Autodesk Inventor part; units mm, degrees
(part 3 of 10)
  spline S18 degree 5 poles (-4.7205, -4.5819) (-4.7206, -4.5819) (-4.7207, -4.582) (-4.7208, -4.5822) (-4.7211, -4.5824) (-4.7215, -4.5828) (-4.7219, -4.5833) (-4.7224, -4.5838) (-4.723, -4.5844) (-4.7236, -4.585) (-4.7242, -4.5857) (-4.7249, -4.5864) (-4.7257, -4.5872) (-4.7265, -4.5881) (-4.7273, -4.589) (-4.7282, -4.59) (-4.7292, -4.5911) (-4.7302, -4.5922) (-4.7312, -4.5933) (-4.7323, -4.5946) (-4.7335, -4.5958) (-4.7346, -4.5972) (-4.7358, -4.5986) (-4.7371, -4.6) (-4.7384, -4.6015) (-4.7397, -4.6031) (-4.7411, -4.6047) (-4.7425, -4.6064) (-4.744, -4.6081) (-4.7455, -4.6099) (-4.747, -4.6117) (-4.7485, -4.6136) (-4.7501, -4.6156) (-4.7518, -4.6176) (-4.7534, -4.6197) (-4.7555, -4.6222) (-4.7576, -4.6248) (-4.7597, -4.6276) (-4.7626, -4.6313) (-4.7663, -4.6361) (-4.7698, -4.6407) (-4.7734, -4.6455) (-4.777, -4.6504) (-4.7812, -4.6561) (-4.7846, -4.6607) (-4.788, -4.6655) (-4.7915, -4.6705) (-4.796, -4.6769) (-4.7992, -4.6815) (-4.8024, -4.6862) (-4.8057, -4.691) (-4.8104, -4.698) (-4.8142, -4.7038) (-4.8181, -4.7097) (-4.822, -4.7157) (-4.827, -4.7234) (-4.8305, -4.729) (-4.834, -4.7346) (-4.8376, -4.7403) (-4.8422, -4.7478) (-4.8458, -4.7537) (-4.8494, -4.7598) (-4.8531, -4.7659) (-4.8584, -4.7748) (-4.8627, -4.7821) (-4.8669, -4.7895) (-4.8712, -4.7971) (-4.8767, -4.8067) (-4.8805, -4.8135) (-4.8843, -4.8204) (-4.8881, -4.8274) (-4.8931, -4.8366) (-4.897, -4.8438) (-4.9008, -4.8511) (-4.9047, -4.8585) (-4.9097, -4.8682) (-4.9136, -4.8758) (-4.9176, -4.8835) (-4.9221, -4.8924) (-4.9265, -4.9014) (-4.9299, -4.9083) (-4.9333, -4.9152) (-4.9384, -4.9257) (-4.9429, -4.9351) (-4.9474, -4.9447) (-4.9519, -4.9544) (-4.9575, -4.9666) (-4.9615, -4.9753) (-4.9654, -4.9841) (-4.9694, -4.9929) (-4.9745, -5.0044) (-4.9784, -5.0135) (-4.9823, -5.0226) (-4.9862, -5.0318) (-4.9918, -5.0451) (-4.9963, -5.0559) (-5.0008, -5.0668) (-5.0052, -5.0778) (-5.0107, -5.0917) (-5.0146, -5.1015) (-5.0185, -5.1114) (-5.0228, -5.1228) (-5.0272, -5.1344) (-5.0305, -5.1431) (-5.0343, -5.1533) (-5.0381, -5.1636) (-5.0413, -5.1725) (-5.0451, -5.183) (-5.0488, -5.1935) (-5.052, -5.2026) (-5.0557, -5.2133) (-5.0594, -5.2241) (-5.0626, -5.2333) (-5.0662, -5.2442) (-5.0699, -5.2552) (-5.073, -5.2647) (-5.0766, -5.2758) (-5.0801, -5.287) (-5.0832, -5.2967) (-5.0867, -5.308) (-5.0903, -5.3194) (-5.0933, -5.3293) (-5.0967, -5.3408) (-5.1002, -5.3525) (-5.1031, -5.3625) (-5.1066, -5.3742) (-5.1099, -5.3861) (-5.1128, -5.3963) (-5.1162, -5.4082) (-5.1195, -5.4203) (-5.1223, -5.4307) (-5.1256, -5.4428) (-5.1288, -5.4551) (-5.1315, -5.4656) (-5.1347, -5.478) (-5.1379, -5.4904) (-5.1406, -5.5012) (-5.1441, -5.5155) (-5.1476, -5.53) (-5.1506, -5.5427) (-5.154, -5.5574) (-5.1574, -5.5721) (-5.1599, -5.5832) (-5.1632, -5.5981) (-5.1665, -5.613) (-5.1693, -5.6262) (-5.1721, -5.6394) (-5.1757, -5.6565) (-5.1784, -5.6699) (-5.181, -5.6833) (-5.1837, -5.6969) (-5.1863, -5.7104) (-5.1881, -5.7202) (-5.1899, -5.7299) (-5.1917, -5.7397) (-5.1935, -5.7496) (-5.1953, -5.7594) (-5.197, -5.7693) (-5.1987, -5.7793) (-5.2004, -5.7892) (-5.2021, -5.7992) (-5.2038, -5.8092) (-5.2054, -5.8193) (-5.207, -5.8294) (-5.2087, -5.8395) (-5.2102, -5.8496) (-5.2118, -5.8598) (-5.2133, -5.87) (-5.2149, -5.8803) (-5.2164, -5.8905) (-5.2178, -5.9008) (-5.2193, -5.9112) (-5.2207, -5.9215) (-5.2222, -5.9319) (-5.2236, -5.9424) (-5.2249, -5.9528) (-5.2263, -5.9633) (-5.2276, -5.9738) (-5.2289, -5.9844) (-5.231, -6.0013) (-5.2327, -6.0161) (-5.2342, -6.0289) (-5.2354, -6.0396) (-5.2363, -6.0482) knots 0 0 0 0 0 0 0.004167 0.008333 0.0125 0.016667 0.020833 0.025 0.029167 0.033333 0.0375 0.041667 0.045833 0.05 0.054167 0.058333 0.0625 0.066667 0.070833 0.075 0.079167 0.083333 0.0875 0.091667 0.095833 0.1 0.104167 0.108333 0.1125 0.116667 0.120833 0.125 0.129167 0.133333 0.1375 0.141667 0.15 0.154167 0.158333 0.170833 0.183333 0.1875 0.191667 0.195833 0.2125 0.216667 0.220833 0.225 0.2375 0.241667 0.245833 0.25 0.266667 0.270833 0.275 0.279167 0.291667 0.295833 0.3 0.304167 0.316667 0.320833 0.325 0.329167 0.345833 0.35 0.354167 0.358333 0.370833 0.375 0.379167 0.383333 0.395833 0.4 0.404167 0.408333 0.420833 0.425 0.429167 0.4375 0.441667 0.445833 0.45 0.466667 0.470833 0.475 0.479167 0.491667 0.495833 0.5 0.504167 0.516667 0.520833 0.525 0.529167 0.545833 0.55 0.554167 0.558333 0.570833 0.575 0.579167 0.5875 0.591667 0.595833 0.604167 0.608333 0.6125 0.620833 0.625 0.629167 0.6375 0.641667 0.645833 0.654167 0.658333 0.6625 0.670833 0.675 0.679167 0.6875 0.691667 0.695833 0.704167 0.708333 0.7125 0.720833 0.725 0.729167 0.7375 0.741667 0.745833 0.754167 0.758333 0.7625 0.770833 0.775 0.779167 0.791667 0.795833 0.8 0.808333 0.8125 0.816667 0.829167 0.833333 0.8375 0.841667 0.854167 0.858333 0.8625 0.866667 0.870833 0.875 0.879167 0.883333 0.8875 0.891667 0.895833 0.9 0.904167 0.908333 0.9125 0.916667 0.920833 0.925 0.929167 0.933333 0.9375 0.941667 0.945833 0.95 0.954167 0.958333 0.9625 0.966667 0.970833 0.975 0.979167 0.983333 1 1 1 1 1 1
  arc A19 (-5.2363, -6.0482) -> (-4.7314, -6.4509) centre (0, 0) ccw
  spline S19 degree 5 poles (-4.7314, -6.4509) (-4.7253, -6.4488) (-4.7171, -6.4459) (-4.707, -6.4424) (-4.6949, -6.4381) (-4.6808, -6.4331) (-4.6708, -6.4295) (-4.6608, -6.4258) (-4.6508, -6.4222) (-4.6409, -6.4186) (-4.631, -6.4149) (-4.6212, -6.4112) (-4.6114, -6.4075) (-4.6016, -6.4038) (-4.5918, -6.4001) (-4.5821, -6.3963) (-4.5724, -6.3926) (-4.5628, -6.3888) (-4.5532, -6.3851) (-4.5436, -6.3813) (-4.534, -6.3775) (-4.5245, -6.3737) (-4.5151, -6.3698) (-4.5056, -6.366) (-4.4962, -6.3621) (-4.4869, -6.3583) (-4.4775, -6.3544) (-4.4682, -6.3505) (-4.459, -6.3466) (-4.4498, -6.3427) (-4.4406, -6.3388) (-4.4277, -6.3333) (-4.415, -6.3277) (-4.4023, -6.3222) (-4.3898, -6.3166) (-4.3737, -6.3094) (-4.3559, -6.3014) (-4.3383, -6.2933) (-4.3209, -6.2852) (-4.3036, -6.277) (-4.2865, -6.2688) (-4.2745, -6.2631) (-4.2627, -6.2573) (-4.2509, -6.2516) (-4.2359, -6.2441) (-4.2243, -6.2383) (-4.2128, -6.2325) (-4.1997, -6.2258) (-4.1867, -6.2191) (-4.177, -6.2141) (-4.1658, -6.2082) (-4.1547, -6.2023) (-4.1452, -6.1972) (-4.1342, -6.1913) (-4.1233, -6.1854) (-4.114, -6.1803) (-4.1032, -6.1744) (-4.0925, -6.1685) (-4.0834, -6.1634) (-4.0728, -6.1574) (-4.0623, -6.1514) (-4.0534, -6.1463) (-4.043, -6.1404) (-4.0328, -6.1344) (-4.024, -6.1292) (-4.0139, -6.1233) (-4.0039, -6.1173) (-3.9953, -6.1121) (-3.9854, -6.1061) (-3.9756, -6.1002) (-3.9673, -6.095) (-3.9576, -6.089) (-3.948, -6.083) (-3.9398, -6.0779) (-3.9317, -6.0727) (-3.9197, -6.065) (-3.9091, -6.0582) (-3.8986, -6.0514) (-3.8882, -6.0445) (-3.8754, -6.036) (-3.8665, -6.03) (-3.8577, -6.0241) (-3.849, -6.0181) (-3.838, -6.0105) (-3.8294, -6.0045) (-3.821, -5.9986) (-3.8126, -5.9927) (-3.8008, -5.9843) (-3.7915, -5.9776) (-3.7823, -5.9708) (-3.7732, -5.9642) (-3.762, -5.9558) (-3.7542, -5.95) (-3.7465, -5.9442) (-3.7389, -5.9384) (-3.7293, -5.931) (-3.7219, -5.9253) (-3.7146, -5.9196) (-3.7074, -5.9139) (-3.6982, -5.9066) (-3.6912, -5.9009) (-3.6842, -5.8953) (-3.6764, -5.8889) (-3.6687, -5.8825) (-3.663, -5.8778) (-3.6564, -5.8723) (-3.6499, -5.8668) (-3.6444, -5.8621) (-3.638, -5.8567) (-3.6318, -5.8513) (-3.6265, -5.8466) (-3.6204, -5.8413) (-3.6144, -5.836) (-3.6093, -5.8315) (-3.6035, -5.8262) (-3.5977, -5.821) (-3.5929, -5.8166) (-3.5873, -5.8114) (-3.5818, -5.8063) (-3.5771, -5.802) (-3.5718, -5.7969) (-3.5665, -5.792) (-3.5621, -5.7877) (-3.557, -5.7828) (-3.552, -5.778) (-3.5478, -5.7738) (-3.5429, -5.7691) (-3.5382, -5.7643) (-3.5342, -5.7603) (-3.5296, -5.7557) (-3.5251, -5.7511) (-3.5214, -5.7472) (-3.517, -5.7427) (-3.5128, -5.7383) (-3.5092, -5.7346) (-3.5052, -5.7302) (-3.5012, -5.726) (-3.4979, -5.7224) (-3.494, -5.7182) (-3.4903, -5.7141) (-3.4872, -5.7107) (-3.4837, -5.7067) (-3.4802, -5.7028) (-3.4773, -5.6995) (-3.474, -5.6958) (-3.4708, -5.6921) (-3.4681, -5.689) (-3.4655, -5.6859) (-3.4622, -5.6819) (-3.4593, -5.6785) (-3.4565, -5.6752) (-3.4539, -5.6719) (-3.4513, -5.6687) (-3.4495, -5.6665) (-3.4478, -5.6644) (-3.4461, -5.6622) (-3.4445, -5.6602) (-3.4429, -5.6581) (-3.4413, -5.6561) (-3.4398, -5.6542) (-3.4383, -5.6523) (-3.4369, -5.6504) (-3.4356, -5.6486) (-3.4342, -5.6469) (-3.433, -5.6452) (-3.4317, -5.6435) (-3.4306, -5.6419) (-3.4294, -5.6404) (-3.4283, -5.6389) (-3.4273, -5.6374) (-3.4263, -5.6361) (-3.4254, -5.6347) (-3.4245, -5.6335) (-3.4236, -5.6322) (-3.4228, -5.6311) (-3.4221, -5.63) (-3.4213, -5.6289) (-3.4207, -5.628) (-3.4201, -5.627) (-3.4195, -5.6262) (-3.419, -5.6254) (-3.4185, -5.6247) (-3.418, -5.624) (-3.4176, -5.6234) (-3.4172, -5.6228) (-3.417, -5.6223) (-3.4168, -5.622) (-3.4166, -5.6218) (-3.4166, -5.6217) knots -1 -1 -1 -1 -1 -1 -0.9875 -0.983333 -0.979167 -0.975 -0.970833 -0.966667 -0.9625 -0.958333 -0.954167 -0.95 -0.945833 -0.941667 -0.9375 -0.933333 -0.929167 -0.925 -0.920833 -0.916667 -0.9125 -0.908333 -0.904167 -0.9 -0.895833 -0.891667 -0.8875 -0.883333 -0.879167 -0.875 -0.870833 -0.866667 -0.854167 -0.85 -0.845833 -0.841667 -0.829167 -0.8125 -0.808333 -0.804167 -0.8 -0.7875 -0.783333 -0.779167 -0.775 -0.7625 -0.758333 -0.754167 -0.745833 -0.741667 -0.7375 -0.729167 -0.725 -0.720833 -0.7125 -0.708333 -0.704167 -0.695833 -0.691667 -0.6875 -0.679167 -0.675 -0.670833 -0.6625 -0.658333 -0.654167 -0.645833 -0.641667 -0.6375 -0.629167 -0.625 -0.620833 -0.6125 -0.608333 -0.604167 -0.6 -0.583333 -0.579167 -0.575 -0.570833 -0.558333 -0.554167 -0.55 -0.545833 -0.533333 -0.529167 -0.525 -0.520833 -0.504167 -0.5 -0.495833 -0.491667 -0.479167 -0.475 -0.470833 -0.466667 -0.454167 -0.45 -0.445833 -0.441667 -0.429167 -0.425 -0.420833 -0.4125 -0.408333 -0.404167 -0.395833 -0.391667 -0.3875 -0.379167 -0.375 -0.370833 -0.3625 -0.358333 -0.354167 -0.345833 -0.341667 -0.3375 -0.329167 -0.325 -0.320833 -0.3125 -0.308333 -0.304167 -0.295833 -0.291667 -0.2875 -0.279167 -0.275 -0.270833 -0.2625 -0.258333 -0.254167 -0.245833 -0.241667 -0.2375 -0.229167 -0.225 -0.220833 -0.2125 -0.208333 -0.204167 -0.195833 -0.191667 -0.1875 -0.179167 -0.175 -0.170833 -0.166667 -0.154167 -0.15 -0.145833 -0.141667 -0.1375 -0.133333 -0.129167 -0.125 -0.120833 -0.116667 -0.1125 -0.108333 -0.104167 -0.1 -0.095833 -0.091667 -0.0875 -0.083333 -0.079167 -0.075 -0.070833 -0.066667 -0.0625 -0.058333 -0.054167 -0.05 -0.045833 -0.041667 -0.0375 -0.033333 -0.029167 -0.025 -0.020833 -0.016667 -0.0125 -0.008333 0 0 0 0 0 0
  line L37 (-3.4166, -5.6217) -> (-3.4162, -5.6212)
  line L38 (-0.6391, -6.5474) -> (-0.639, -6.5467)
  line L39 (-0.639, -6.5467) -> (-0.5586, -5.7228)
  arc A20 (-0.5586, -5.7228) -> (0.5586, -5.7228) centre (0, 0) ccw
  line L40 (0.5586, -5.7228) -> (0.639, -6.5467)
  line L41 (0.639, -6.5467) -> (0.6391, -6.5474)
  spline S20 degree 5 poles (0.6391, -6.5474) (0.6391, -6.5475) (0.6391, -6.5476) (0.6391, -6.5478) (0.6391, -6.5482) (0.6392, -6.5488) (0.6393, -6.5494) (0.6394, -6.5501) (0.6395, -6.5509) (0.6396, -6.5517) (0.6397, -6.5527) (0.6399, -6.5537) (0.64, -6.5548) (0.6402, -6.556) (0.6404, -6.5572) (0.6406, -6.5585) (0.6408, -6.5599) (0.6411, -6.5614) (0.6413, -6.5629) (0.6416, -6.5645) (0.6419, -6.5662) (0.6422, -6.568) (0.6425, -6.5698) (0.6429, -6.5717) (0.6433, -6.5736) (0.6437, -6.5756) (0.6441, -6.5777) (0.6445, -6.5799) (0.6449, -6.5821) (0.6454, -6.5844) (0.6459, -6.5867) (0.6464, -6.5891) (0.6469, -6.5916) (0.6475, -6.5941) (0.6481, -6.5967) (0.6488, -6.5999) (0.6496, -6.6032) (0.6504, -6.6065) (0.6515, -6.6111) (0.6529, -6.6171) (0.6543, -6.6226) (0.6558, -6.6284) (0.6574, -6.6343) (0.6592, -6.6411) (0.6608, -6.6466) (0.6624, -6.6523) (0.6641, -6.6582) (0.6663, -6.6657) (0.6679, -6.671) (0.6696, -6.6765) (0.6713, -6.682) (0.6738, -6.6901) (0.676, -6.6966) (0.6781, -6.7034) (0.6804, -6.7102) (0.6834, -6.7189) (0.6855, -6.7251) (0.6877, -6.7313) (0.69, -6.7377) (0.6929, -6.746) (0.6953, -6.7525) (0.6978, -6.7591) (0.7003, -6.7658) (0.704, -6.7755) (0.707, -6.7834) (0.7101, -6.7913) (0.7133, -6.7994) (0.7175, -6.8096) (0.7204, -6.8169) (0.7234, -6.8242) (0.7265, -6.8315) (0.7306, -6.8411) (0.7338, -6.8486) (0.7371, -6.8562) (0.7405, -6.8639) (0.7454, -6.8749) (0.7494, -6.8839) (0.7535, -6.8929) (0.7578, -6.902) (0.7631, -6.9135) (0.767, -6.9216) (0.7709, -6.9297) (0.7749, -6.938) (0.7801, -6.9486) (0.7842, -6.957) (0.7884, -6.9654) (0.7927, -6.9738) (0.7983, -6.9848) (0.8027, -6.9933) (0.8072, -7.002) (0.8124, -7.0119) (0.8177, -7.0219) (0.8218, -7.0294) (0.8266, -7.0382) (0.8314, -7.0471) (0.8356, -7.0548) (0.8406, -7.0637) (0.8456, -7.0727) (0.85, -7.0805) (0.8552, -7.0896) (0.8605, -7.0987) (0.865, -7.1066) (0.8704, -7.1158) (0.8758, -7.125) (0.8806, -7.133) (0.8862, -7.1423) (0.8918, -7.1517) (0.8967, -7.1597) (0.9025, -7.1692) (0.9084, -7.1786) (0.9134, -7.1868) (0.9194, -7.1963) (0.9255, -7.2059) (0.9307, -7.2141) (0.9369, -7.2238) (0.9432, -7.2334) (0.9486, -7.2417) (0.955, -7.2515) (0.9615, -7.2612) (0.9671, -7.2696) (0.9737, -7.2794) (0.9804, -7.2893) (0.9861, -7.2978) (0.993, -7.3077) (0.9998, -7.3176) (1.0058, -7.3261) (1.0128, -7.3361) (1.0199, -7.3461) (1.026, -7.3547) (1.0333, -7.3648) (1.0406, -7.3748) (1.0469, -7.3835) (1.0543, -7.3936) (1.0618, -7.4038) (1.0683, -7.4125) (1.0759, -7.4227) (1.0836, -7.4329) (1.0903, -7.4417) (1.0981, -7.4519) (1.1061, -7.4622) (1.1129, -7.471) (1.121, -7.4813) (1.1291, -7.4916) (1.1361, -7.5005) (1.1432, -7.5093) (1.1527, -7.5212) (1.1611, -7.5316) (1.1696, -7.542) (1.1794, -7.5539) (1.1893, -7.5658) (1.1967, -7.5748) (1.2043, -7.5837) (1.2131, -7.5942) (1.2207, -7.6032) (1.2297, -7.6137) (1.2388, -7.6242) (1.2479, -7.6347) (1.2558, -7.6437) (1.2637, -7.6528) (1.2704, -7.6603) (1.2771, -7.6678) (1.2838, -7.6754) (1.2905, -7.6829) (1.2973, -7.6905) (1.3042, -7.698) (1.311, -7.7056) (1.318, -7.7132) (1.3249, -7.7207) (1.3319, -7.7283) (1.3389, -7.7359) (1.346, -7.7434) (1.3531, -7.751) (1.3602, -7.7586) (1.3674, -7.7662) (1.3746, -7.7738) (1.3818, -7.7813) (1.3891, -7.7889) (1.3964, -7.7965) (1.4038, -7.8041) (1.4111, -7.8117) (1.4186, -7.8193) (1.4305, -7.8315) (1.4411, -7.8421) (1.4502, -7.8512) (1.4578, -7.8588) (1.4639, -7.8649) knots 0 0 0 0 0 0 0.004167 0.008333 0.0125 0.016667 0.020833 0.025 0.029167 0.033333 0.0375 0.041667 0.045833 0.05 0.054167 0.058333 0.0625 0.066667 0.070833 0.075 0.079167 0.083333 0.0875 0.091667 0.095833 0.1 0.104167 0.108333 0.1125 0.116667 0.120833 0.125 0.129167 0.133333 0.1375 0.141667 0.15 0.154167 0.158333 0.170833 0.183333 0.1875 0.191667 0.195833 0.2125 0.216667 0.220833 0.225 0.2375 0.241667 0.245833 0.25 0.266667 0.270833 0.275 0.279167 0.291667 0.295833 0.3 0.304167 0.316667 0.320833 0.325 0.329167 0.345833 0.35 0.354167 0.358333 0.370833 0.375 0.379167 0.383333 0.395833 0.4 0.404167 0.408333 0.425 0.429167 0.433333 0.4375 0.45 0.454167 0.458333 0.4625 0.475 0.479167 0.483333 0.4875 0.5 0.504167 0.508333 0.516667 0.520833 0.525 0.533333 0.5375 0.541667 0.55 0.554167 0.558333 0.566667 0.570833 0.575 0.583333 0.5875 0.591667 0.6 0.604167 0.608333 0.616667 0.620833 0.625 0.633333 0.6375 0.641667 0.65 0.654167 0.658333 0.666667 0.670833 0.675 0.683333 0.6875 0.691667 0.7 0.704167 0.708333 0.716667 0.720833 0.725 0.733333 0.7375 0.741667 0.75 0.754167 0.758333 0.766667 0.770833 0.775 0.783333 0.7875 0.791667 0.8 0.804167 0.808333 0.8125 0.825 0.829167 0.833333 0.841667 0.845833 0.85 0.854167 0.8625 0.866667 0.875 0.879167 0.883333 0.8875 0.891667 0.895833 0.9 0.904167 0.908333 0.9125 0.916667 0.920833 0.925 0.929167 0.933333 0.9375 0.941667 0.945833 0.95 0.954167 0.958333 0.9625 0.966667 0.970833 0.975 0.979167 0.983333 1 1 1 1 1 1
  arc A21 (1.4639, -7.8649) -> (2.0935, -7.7212) centre (0, 0) ccw
  spline S21 degree 5 poles (2.0935, -7.7212) (2.0957, -7.7151) (2.0986, -7.707) (2.1021, -7.6968) (2.1063, -7.6847) (2.1112, -7.6705) (2.1146, -7.6605) (2.118, -7.6504) (2.1213, -7.6403) (2.1247, -7.6303) (2.128, -7.6203) (2.1312, -7.6103) (2.1345, -7.6003) (2.1377, -7.5904) (2.1408, -7.5804) (2.144, -7.5705) (2.1471, -7.5606) (2.1501, -7.5507) (2.1532, -7.5408) (2.1562, -7.531) (2.1592, -7.5211) (2.1621, -7.5113) (2.165, -7.5015) (2.1679, -7.4918) (2.1708, -7.482) (2.1736, -7.4723) (2.1764, -7.4626) (2.1791, -7.4529) (2.1818, -7.4432) (2.1845, -7.4336) (2.1877, -7.422) (2.1909, -7.4105) (2.194, -7.399) (2.197, -7.3875) (2.2011, -7.3723) (2.2045, -7.359) (2.2079, -7.3458) (2.2112, -7.3326) (2.2154, -7.3157) (2.2186, -7.3026) (2.2217, -7.2895) (2.2248, -7.2765) (2.2291, -7.258) (2.2324, -7.2433) (2.2357, -7.2286) (2.2388, -7.214) (2.2427, -7.1958) (2.2454, -7.1832) (2.248, -7.1706) (2.2505, -7.158) (2.2537, -7.1419) (2.2561, -7.1295) (2.2584, -7.1171) (2.2607, -7.1048) (2.2639, -7.0872) (2.2664, -7.0733) (2.2688, -7.0594) (2.2711, -7.0456) (2.2739, -7.0284) (2.2758, -7.0165) (2.2776, -7.0046) (2.2794, -6.9928) (2.2817, -6.9777) (2.2833, -6.966) (2.285, -6.9543) (2.2868, -6.9411) (2.2885, -6.928) (2.2897, -6.9182) (2.2911, -6.9068) (2.2925, -6.8954) (2.2936, -6.8858) (2.2949, -6.8746) (2.2961, -6.8634) (2.2971, -6.8539) (2.2983, -6.8429) (2.2993, -6.8319) (2.3002, -6.8226) (2.3012, -6.8117) (2.3022, -6.801) (2.303, -6.7918) (2.3038, -6.7811) (2.3046, -6.7706) (2.3053, -6.7615) (2.3061, -6.7511) (2.3067, -6.7407) (2.3073, -6.7318) (2.3079, -6.7216) (2.3085, -6.7114) (2.3089, -6.7027) (2.3094, -6.6927) (2.3099, -6.6827) (2.3102, -6.6742) (2.3106, -6.6644) (2.3109, -6.6546) (2.3112, -6.6463) (2.3114, -6.6367) (2.3116, -6.6271) (2.3118, -6.619) (2.3119, -6.6096) (2.312, -6.6003) (2.3121, -6.5923) (2.3121, -6.5832) (2.3121, -6.5741) (2.3121, -6.5663) (2.3121, -6.5574) (2.312, -6.5485) (2.3118, -6.541) (2.3117, -6.5323) (2.3115, -6.5237) (2.3113, -6.5163) (2.3111, -6.5078) (2.3108, -6.4995) (2.3105, -6.4924) (2.3102, -6.4841) (2.3098, -6.476) (2.3095, -6.4691) (2.309, -6.4611) (2.3086, -6.4532) (2.3082, -6.4466) (2.3077, -6.4388) (2.3072, -6.4312) (2.3067, -6.4248) (2.3061, -6.4173) (2.3055, -6.41) (2.305, -6.4038) (2.3044, -6.3966) (2.3037, -6.3895) (2.3031, -6.3835) (2.3025, -6.3766) (2.3017, -6.3698) (2.3011, -6.3641) (2.3004, -6.3575) (2.2996, -6.3509) (2.299, -6.3454) (2.2982, -6.3391) (2.2974, -6.3329) (2.2967, -6.3277) (2.2958, -6.3216) (2.295, -6.3157) (2.2943, -6.3107) (2.2934, -6.305) (2.2926, -6.2994) (2.2918, -6.2947) (2.2909, -6.2893) (2.2901, -6.284) (2.2893, -6.2795) (2.2884, -6.2744) (2.2875, -6.2695) (2.2867, -6.2653) (2.286, -6.2612) (2.2852, -6.2572) (2.2843, -6.2526) (2.2834, -6.2482) (2.2825, -6.2439) (2.2816, -6.2397) (2.2808, -6.2356) (2.2801, -6.2328) (2.2795, -6.23) (2.2789, -6.2273) (2.2783, -6.2246) (2.2777, -6.222) (2.2771, -6.2195) (2.2765, -6.2171) (2.2759, -6.2147) (2.2754, -6.2123) (2.2748, -6.2101) (2.2742, -6.2079) (2.2737, -6.2058) (2.2732, -6.2037) (2.2726, -6.2017) (2.2721, -6.1998) (2.2716, -6.198) (2.2711, -6.1962) (2.2706, -6.1945) (2.2702, -6.1928) (2.2697, -6.1913) (2.2693, -6.1898) (2.2689, -6.1883) (2.2685, -6.187) (2.2681, -6.1857) (2.2677, -6.1845) (2.2674, -6.1834) (2.267, -6.1823) (2.2667, -6.1813) (2.2664, -6.1804) (2.2662, -6.1796) (2.2659, -6.1788) (2.2657, -6.1782) (2.2654, -6.1774) (2.2653, -6.1769) (2.2652, -6.1766) (2.2651, -6.1764) (2.265, -6.1763) knots -1 -1 -1 -1 -1 -1 -0.9875 -0.983333 -0.979167 -0.975 -0.970833 -0.966667 -0.9625 -0.958333 -0.954167 -0.95 -0.945833 -0.941667 -0.9375 -0.933333 -0.929167 -0.925 -0.920833 -0.916667 -0.9125 -0.908333 -0.904167 -0.9 -0.895833 -0.891667 -0.8875 -0.883333 -0.879167 -0.875 -0.870833 -0.8625 -0.858333 -0.854167 -0.85 -0.8375 -0.833333 -0.829167 -0.825 -0.8125 -0.808333 -0.804167 -0.8 -0.783333 -0.779167 -0.775 -0.770833 -0.758333 -0.754167 -0.75 -0.745833 -0.733333 -0.729167 -0.725 -0.720833 -0.704167 -0.7 -0.695833 -0.691667 -0.679167 -0.675 -0.670833 -0.666667 -0.654167 -0.65 -0.645833 -0.6375 -0.633333 -0.629167 -0.620833 -0.616667 -0.6125 -0.604167 -0.6 -0.595833 -0.5875 -0.583333 -0.579167 -0.570833 -0.566667 -0.5625 -0.554167 -0.55 -0.545833 -0.5375 -0.533333 -0.529167 -0.520833 -0.516667 -0.5125 -0.504167 -0.5 -0.495833 -0.4875 -0.483333 -0.479167 -0.470833 -0.466667 -0.4625 -0.454167 -0.45 -0.445833 -0.4375 -0.433333 -0.429167 -0.420833 -0.416667 -0.4125 -0.404167 -0.4 -0.395833 -0.3875 -0.383333 -0.379167 -0.370833 -0.366667 -0.3625 -0.354167 -0.35 -0.345833 -0.3375 -0.333333 -0.329167 -0.320833 -0.316667 -0.3125 -0.304167 -0.3 -0.295833 -0.2875 -0.283333 -0.279167 -0.270833 -0.266667 -0.2625 -0.254167 -0.25 -0.245833 -0.2375 -0.233333 -0.229167 -0.220833 -0.216667 -0.2125 -0.204167 -0.2 -0.195833 -0.1875 -0.183333 -0.179167 -0.175 -0.170833 -0.158333 -0.154167 -0.15 -0.145833 -0.141667 -0.1375 -0.133333 -0.129167 -0.125 -0.120833 -0.116667 -0.1125 -0.108333 -0.104167 -0.1 -0.095833 -0.091667 -0.0875 -0.083333 -0.079167 -0.075 -0.070833 -0.066667 -0.0625 -0.058333 -0.054167 -0.05 -0.045833 -0.041667 -0.0375 -0.033333 -0.029167 -0.025 -0.020833 -0.016667 -0.0125 -0.008333 0 0 0 0 0 0
  line L42 (2.265, -6.1763) -> (2.2648, -6.1757)
  line L43 (2.2648, -6.1757) -> (1.9798, -5.3984)
  arc A22 (1.9798, -5.3984) -> (2.9863, -4.9137) centre (0, 0) ccw
  line L44 (4.7205, -4.5819) -> (4.72, -4.5814)
  line L45 (4.72, -4.5814) -> (4.126, -4.0048)
  spline S22 degree 5 poles (5.2363, -6.0482) (5.2356, -6.0418) (5.2347, -6.0332) (5.2335, -6.0225) (5.232, -6.0098) (5.2302, -5.9949) (5.2289, -5.9844) (5.2276, -5.9738) (5.2263, -5.9633) (5.2249, -5.9528) (5.2236, -5.9424) (5.2222, -5.9319) (5.2207, -5.9215) (5.2193, -5.9112) (5.2178, -5.9008) (5.2164, -5.8905) (5.2149, -5.8803) (5.2133, -5.87) (5.2118, -5.8598) (5.2102, -5.8496) (5.2087, -5.8395) (5.207, -5.8294) (5.2054, -5.8193) (5.2038, -5.8092) (5.2021, -5.7992) (5.2004, -5.7892) (5.1987, -5.7793) (5.197, -5.7693) (5.1953, -5.7594) (5.1935, -5.7496) (5.1917, -5.7397) (5.1892, -5.726) (5.1866, -5.7124) (5.1841, -5.6988) (5.1814, -5.6853) (5.178, -5.668) (5.1741, -5.6489) (5.1702, -5.6299) (5.1661, -5.6111) (5.162, -5.5925) (5.1578, -5.5739) (5.1549, -5.561) (5.1519, -5.5482) (5.1489, -5.5355) (5.145, -5.5191) (5.1419, -5.5065) (5.1388, -5.494) (5.1352, -5.4798) (5.1315, -5.4656) (5.1288, -5.4551) (5.1256, -5.4428) (5.1223, -5.4307) (5.1195, -5.4203) (5.1162, -5.4082) (5.1128, -5.3963) (5.1099, -5.3861) (5.1066, -5.3742) (5.1031, -5.3625) (5.1002, -5.3525) (5.0967, -5.3408) (5.0933, -5.3293) (5.0903, -5.3194) (5.0867, -5.308) (5.0832, -5.2967) (5.0801, -5.287) (5.0771, -5.2774) (5.073, -5.2647) (5.0693, -5.2536) (5.0657, -5.2427) (5.0615, -5.2302) (5.0573, -5.2179) (5.0541, -5.2087) (5.0504, -5.1981) (5.0467, -5.1875) (5.0434, -5.1785) (5.0397, -5.1681) (5.0359, -5.1577) (5.0327, -5.1489) (5.0288, -5.1387) (5.025, -5.1286) (5.0217, -5.12) (5.0179, -5.11) (5.014, -5.1001) (5.0107, -5.0917) (5.0069, -5.082) (5.003, -5.0723) (4.9996, -5.0641) (4.9957, -5.0546) (4.9918, -5.0452) (4.9885, -5.0372) (4.9846, -5.0279) (4.9806, -5.0187) (4.9773, -5.0109) (4.9733, -5.0019) (4.9694, -4.9929) (4.966, -4.9853) (4.9621, -4.9766) (4.9581, -4.9679) (4.9547, -4.9605) (4.9508, -4.9519) (4.9468, -4.9435) (4.9434, -4.9363) (4.9395, -4.928) (4.9356, -4.9198) (4.9322, -4.9129) (4.9282, -4.9048) (4.9243, -4.8969) (4.9209, -4.8902) (4.917, -4.8824) (4.9131, -4.8747) (4.9097, -4.8682) (4.9058, -4.8606) (4.9019, -4.8532) (4.8986, -4.8469) (4.8947, -4.8397) (4.8909, -4.8325) (4.8876, -4.8264) (4.8837, -4.8194) (4.8799, -4.8125) (4.8767, -4.8067) (4.8729, -4.7999) (4.8691, -4.7933) (4.8659, -4.7877) (4.8621, -4.7812) (4.8584, -4.7749) (4.8552, -4.7695) (4.8515, -4.7633) (4.8479, -4.7572) (4.8448, -4.752) (4.8412, -4.7461) (4.8376, -4.7403) (4.8345, -4.7354) (4.831, -4.7298) (4.8275, -4.7242) (4.8245, -4.7196) (4.821, -4.7142) (4.8176, -4.709) (4.8147, -4.7045) (4.8113, -4.6995) (4.808, -4.6945) (4.8052, -4.6903) (4.8019, -4.6855) (4.7987, -4.6808) (4.796, -4.6769) (4.7929, -4.6724) (4.7898, -4.668) (4.7872, -4.6644) (4.7846, -4.6608) (4.7808, -4.6555) (4.7774, -4.6509) (4.7742, -4.6465) (4.771, -4.6423) (4.7679, -4.6382) (4.766, -4.6357) (4.7637, -4.6327) (4.7615, -4.6299) (4.7593, -4.6271) (4.7572, -4.6244) (4.7551, -4.6218) (4.7534, -4.6197) (4.7518, -4.6176) (4.7501, -4.6156) (4.7485, -4.6136) (4.747, -4.6117) (4.7455, -4.6099) (4.744, -4.6081) (4.7425, -4.6064) (4.7411, -4.6047) (4.7397, -4.6031) (4.7384, -4.6015) (4.7371, -4.6) (4.7358, -4.5986) (4.7346, -4.5972) (4.7335, -4.5958) (4.7323, -4.5946) (4.7312, -4.5933) (4.7302, -4.5922) (4.7292, -4.5911) (4.7282, -4.59) (4.7273, -4.589) (4.7265, -4.5881) (4.7257, -4.5872) (4.7249, -4.5864) (4.7242, -4.5857) (4.7236, -4.585) (4.723, -4.5844) (4.7224, -4.5838) (4.7219, -4.5833) (4.7214, -4.5827) (4.721, -4.5824) (4.7208, -4.5821) (4.7206, -4.582) (4.7205, -4.5819) knots -1 -1 -1 -1 -1 -1 -0.9875 -0.983333 -0.979167 -0.975 -0.970833 -0.966667 -0.9625 -0.958333 -0.954167 -0.95 -0.945833 -0.941667 -0.9375 -0.933333 -0.929167 -0.925 -0.920833 -0.916667 -0.9125 -0.908333 -0.904167 -0.9 -0.895833 -0.891667 -0.8875 -0.883333 -0.879167 -0.875 -0.870833 -0.866667 -0.854167 -0.85 -0.845833 -0.841667 -0.829167 -0.8125 -0.808333 -0.804167 -0.8 -0.7875 -0.783333 -0.779167 -0.775 -0.7625 -0.758333 -0.754167 -0.745833 -0.741667 -0.7375 -0.729167 -0.725 -0.720833 -0.7125 -0.708333 -0.704167 -0.695833 -0.691667 -0.6875 -0.679167 -0.675 -0.670833 -0.6625 -0.658333 -0.654167 -0.65 -0.6375 -0.633333 -0.629167 -0.620833 -0.616667 -0.6125 -0.604167 -0.6 -0.595833 -0.5875 -0.583333 -0.579167 -0.570833 -0.566667 -0.5625 -0.554167 -0.55 -0.545833 -0.5375 -0.533333 -0.529167 -0.520833 -0.516667 -0.5125 -0.504167 -0.5 -0.495833 -0.4875 -0.483333 -0.479167 -0.470833 -0.466667 -0.4625 -0.454167 -0.45 -0.445833 -0.4375 -0.433333 -0.429167 -0.420833 -0.416667 -0.4125 -0.404167 -0.4 -0.395833 -0.3875 -0.383333 -0.379167 -0.370833 -0.366667 -0.3625 -0.354167 -0.35 -0.345833 -0.3375 -0.333333 -0.329167 -0.320833 -0.316667 -0.3125 -0.304167 -0.3 -0.295833 -0.2875 -0.283333 -0.279167 -0.270833 -0.266667 -0.2625 -0.254167 -0.25 -0.245833 -0.2375 -0.233333 -0.229167 -0.220833 -0.216667 -0.2125 -0.204167 -0.2 -0.195833 -0.191667 -0.175 -0.170833 -0.166667 -0.1625 -0.158333 -0.154167 -0.145833 -0.141667 -0.1375 -0.133333 -0.129167 -0.125 -0.120833 -0.116667 -0.1125 -0.108333 -0.104167 -0.1 -0.095833 -0.091667 -0.0875 -0.083333 -0.079167 -0.075 -0.070833 -0.066667 -0.0625 -0.058333 -0.054167 -0.05 -0.045833 -0.041667 -0.0375 -0.033333 -0.029167 -0.025 -0.020833 -0.016667 -0.0125 -0.008333 0 0 0 0 0 0
  arc A23 (4.7314, -6.4509) -> (5.2363, -6.0482) centre (0, 0) ccw
  line L46 (3.4162, -5.6212) -> (3.4166, -5.6217)
  line L47 (2.9863, -4.9137) -> (3.4162, -5.6212)
  spline S23 degree 5 poles (3.4166, -5.6217) (3.4166, -5.6218) (3.4167, -5.6219) (3.4168, -5.6221) (3.417, -5.6224) (3.4173, -5.6229) (3.4176, -5.6234) (3.418, -5.624) (3.4185, -5.6247) (3.419, -5.6254) (3.4195, -5.6262) (3.4201, -5.627) (3.4207, -5.628) (3.4213, -5.6289) (3.4221, -5.63) (3.4228, -5.6311) (3.4236, -5.6322) (3.4245, -5.6335) (3.4254, -5.6347) (3.4263, -5.6361) (3.4273, -5.6374) (3.4283, -5.6389) (3.4294, -5.6404) (3.4306, -5.6419) (3.4317, -5.6435) (3.433, -5.6452) (3.4342, -5.6469) (3.4356, -5.6486) (3.4369, -5.6504) (3.4383, -5.6523) (3.4398, -5.6542) (3.4413, -5.6561) (3.4429, -5.6581) (3.4445, -5.6602) (3.4464, -5.6627) (3.4485, -5.6652) (3.4506, -5.6678) (3.4542, -5.6723) (3.4581, -5.677) (3.4621, -5.6819) (3.4664, -5.6869) (3.4708, -5.6921) (3.474, -5.6958) (3.4773, -5.6995) (3.4802, -5.7028) (3.4837, -5.7067) (3.4872, -5.7107) (3.4903, -5.7141) (3.494, -5.7182) (3.4979, -5.7224) (3.5012, -5.726) (3.5052, -5.7302) (3.5092, -5.7346) (3.5128, -5.7383) (3.517, -5.7427) (3.5214, -5.7472) (3.5251, -5.7511) (3.5296, -5.7557) (3.5342, -5.7603) (3.5382, -5.7643) (3.5429, -5.7691) (3.5478, -5.7738) (3.552, -5.778) (3.557, -5.7828) (3.5621, -5.7877) (3.5665, -5.792) (3.5718, -5.7969) (3.5771, -5.802) (3.5818, -5.8063) (3.5873, -5.8114) (3.5929, -5.8166) (3.5977, -5.821) (3.6035, -5.8262) (3.6093, -5.8315) (3.6144, -5.836) (3.6204, -5.8413) (3.6265, -5.8466) (3.6318, -5.8513) (3.638, -5.8567) (3.6444, -5.8621) (3.6499, -5.8668) (3.6564, -5.8723) (3.663, -5.8778) (3.6687, -5.8825) (3.6754, -5.8881) (3.6823, -5.8937) (3.6882, -5.8985) (3.6952, -5.9041) (3.7023, -5.9098) (3.7084, -5.9147) (3.7156, -5.9204) (3.723, -5.9261) (3.7293, -5.931) (3.7368, -5.9368) (3.7444, -5.9426) (3.7509, -5.9475) (3.7586, -5.9533) (3.7664, -5.9592) (3.7732, -5.9642) (3.7811, -5.97) (3.7892, -5.9759) (3.7961, -5.9809) (3.8043, -5.9868) (3.8126, -5.9927) (3.8198, -5.9978) (3.8282, -6.0037) (3.8367, -6.0096) (3.8441, -6.0147) (3.8528, -6.0207) (3.8615, -6.0266) (3.8691, -6.0317) (3.878, -6.0377) (3.887, -6.0437) (3.8947, -6.0488) (3.9039, -6.0548) (3.9131, -6.0608) (3.921, -6.0659) (3.9304, -6.0719) (3.9398, -6.0779) (3.948, -6.083) (3.9576, -6.089) (3.9673, -6.095) (3.9756, -6.1002) (3.984, -6.1053) (3.9967, -6.113) (4.0081, -6.1198) (4.0197, -6.1267) (4.0313, -6.1335) (4.046, -6.1421) (4.0563, -6.148) (4.0668, -6.154) (4.0788, -6.1608) (4.091, -6.1676) (4.1001, -6.1727) (4.1109, -6.1786) (4.1217, -6.1846) (4.1311, -6.1896) (4.142, -6.1956) (4.1531, -6.2015) (4.1626, -6.2065) (4.1738, -6.2124) (4.1851, -6.2183) (4.1948, -6.2233) (4.2062, -6.2291) (4.2177, -6.235) (4.2276, -6.24) (4.2392, -6.2458) (4.2509, -6.2516) (4.261, -6.2565) (4.2712, -6.2615) (4.283, -6.2672) (4.2933, -6.2721) (4.3036, -6.277) (4.3157, -6.2827) (4.3279, -6.2884) (4.3383, -6.2933) (4.3506, -6.2989) (4.363, -6.3046) (4.3737, -6.3094) (4.3844, -6.3142) (4.3987, -6.3206) (4.4114, -6.3261) (4.4241, -6.3317) (4.4369, -6.3372) (4.4498, -6.3427) (4.459, -6.3466) (4.4682, -6.3505) (4.4775, -6.3544) (4.4869, -6.3583) (4.4962, -6.3621) (4.5056, -6.366) (4.5151, -6.3698) (4.5245, -6.3737) (4.534, -6.3775) (4.5436, -6.3813) (4.5532, -6.3851) (4.5628, -6.3888) (4.5724, -6.3926) (4.5821, -6.3963) (4.5918, -6.4001) (4.6016, -6.4038) (4.6114, -6.4075) (4.6212, -6.4112) (4.631, -6.4149) (4.6409, -6.4186) (4.6508, -6.4222) (4.6608, -6.4258) (4.6708, -6.4295) (4.6868, -6.4352) (4.7009, -6.4403) (4.7131, -6.4445) (4.7232, -6.4481) (4.7314, -6.4509) knots 0 0 0 0 0 0 0.004167 0.008333 0.0125 0.016667 0.020833 0.025 0.029167 0.033333 0.0375 0.041667 0.045833 0.05 0.054167 0.058333 0.0625 0.066667 0.070833 0.075 0.079167 0.083333 0.0875 0.091667 0.095833 0.1 0.104167 0.108333 0.1125 0.116667 0.120833 0.125 0.129167 0.133333 0.1375 0.145833 0.15 0.154167 0.175 0.179167 0.1875 0.191667 0.195833 0.204167 0.208333 0.2125 0.220833 0.225 0.229167 0.2375 0.241667 0.245833 0.254167 0.258333 0.2625 0.270833 0.275 0.279167 0.2875 0.291667 0.295833 0.304167 0.308333 0.3125 0.320833 0.325 0.329167 0.3375 0.341667 0.345833 0.354167 0.358333 0.3625 0.370833 0.375 0.379167 0.3875 0.391667 0.395833 0.404167 0.408333 0.4125 0.420833 0.425 0.429167 0.4375 0.441667 0.445833 0.454167 0.458333 0.4625 0.470833 0.475 0.479167 0.4875 0.491667 0.495833 0.504167 0.508333 0.5125 0.520833 0.525 0.529167 0.5375 0.541667 0.545833 0.554167 0.558333 0.5625 0.570833 0.575 0.579167 0.5875 0.591667 0.595833 0.604167 0.608333 0.6125 0.620833 0.625 0.629167 0.6375 0.641667 0.645833 0.65 0.666667 0.670833 0.675 0.679167 0.691667 0.695833 0.7 0.708333 0.7125 0.716667 0.725 0.729167 0.733333 0.741667 0.745833 0.75 0.758333 0.7625 0.766667 0.775 0.779167 0.783333 0.791667 0.795833 0.8 0.804167 0.8125 0.816667 0.820833 0.829167 0.833333 0.8375 0.845833 0.85 0.854167 0.858333 0.870833 0.875 0.879167 0.883333 0.8875 0.891667 0.895833 0.9 0.904167 0.908333 0.9125 0.916667 0.920833 0.925 0.929167 0.933333 0.9375 0.941667 0.945833 0.95 0.954167 0.958333 0.9625 0.966667 0.970833 0.975 0.979167 0.983333 1 1 1 1 1 1
  arc A24 (4.8225, 3.1314) -> (4.126, 4.0048) centre (0, 0) ccw
  line L48 (5.5174, 3.5826) -> (5.5168, 3.5822)
  line L49 (5.5168, 3.5822) -> (4.8225, 3.1314)
  spline S24 degree 5 poles (7.0618, 3.7592) (7.0553, 3.7599) (7.0468, 3.7609) (7.0361, 3.7621) (7.0233, 3.7635) (7.0084, 3.7651) (6.9979, 3.7662) (6.9873, 3.7673) (6.9767, 3.7683) (6.9662, 3.7693) (6.9557, 3.7703) (6.9452, 3.7713) (6.9348, 3.7722) (6.9244, 3.7731) (6.914, 3.774) (6.9036, 3.7748) (6.8933, 3.7756) (6.8829, 3.7764) (6.8726, 3.7772) (6.8624, 3.7779) (6.8521, 3.7787) (6.8419, 3.7793) (6.8317, 3.78) (6.8215, 3.7806) (6.8114, 3.7812) (6.8013, 3.7818) (6.7912, 3.7824) (6.7811, 3.7829) (6.7711, 3.7834) (6.7611, 3.7839) (6.7511, 3.7843) (6.7372, 3.7849) (6.7233, 3.7855) (6.7095, 3.786) (6.6957, 3.7864) (6.6781, 3.7869) (6.6605, 3.7873) (6.6431, 3.7877) (6.6258, 3.7879) (6.6085, 3.7881) (6.5914, 3.7882) (6.5781, 3.7882) (6.5649, 3.7882) (6.5518, 3.7881) (6.5331, 3.788) (6.5182, 3.7878) (6.5034, 3.7875) (6.4887, 3.7872) (6.4705, 3.7867) (6.4578, 3.7863) (6.4451, 3.7858) (6.4325, 3.7854) (6.4164, 3.7847) (6.404, 3.7841) (6.3916, 3.7835) (6.3793, 3.7828) (6.3618, 3.7818) (6.3479, 3.781) (6.3342, 3.7801) (6.3205, 3.7791) (6.3035, 3.7778) (6.2916, 3.7769) (6.2799, 3.7759) (6.2682, 3.7749) (6.2533, 3.7735) (6.2417, 3.7724) (6.2303, 3.7713) (6.2173, 3.7699) (6.2044, 3.7685) (6.1947, 3.7675) (6.1836, 3.7662) (6.1725, 3.7649) (6.1631, 3.7637) (6.1521, 3.7623) (6.1412, 3.7609) (6.132, 3.7597) (6.1212, 3.7582) (6.1106, 3.7568) (6.1015, 3.7555) (6.091, 3.7539) (6.0805, 3.7523) (6.0716, 3.751) (6.0613, 3.7493) (6.0511, 3.7477) (6.0424, 3.7462) (6.0323, 3.7445) (6.0223, 3.7428) (6.0138, 3.7413) (6.004, 3.7395) (5.9942, 3.7377) (5.9859, 3.7361) (5.9763, 3.7343) (5.9667, 3.7324) (5.9586, 3.7308) (5.9493, 3.7289) (5.94, 3.727) (5.9321, 3.7253) (5.9229, 3.7233) (5.9139, 3.7214) (5.9062, 3.7196) (5.8973, 3.7176) (5.8885, 3.7156) (5.881, 3.7138) (5.8723, 3.7118) (5.8638, 3.7097) (5.8565, 3.7079) (5.8481, 3.7058) (5.8398, 3.7037) (5.8328, 3.7019) (5.8246, 3.6997) (5.8166, 3.6976) (5.8098, 3.6957) (5.8019, 3.6935) (5.7941, 3.6914) (5.7875, 3.6895) (5.7799, 3.6873) (5.7724, 3.6851) (5.766, 3.6832) (5.7587, 3.681) (5.7514, 3.6788) (5.7453, 3.6769) (5.7382, 3.6747) (5.7313, 3.6725) (5.7254, 3.6706) (5.7186, 3.6684) (5.7119, 3.6662) (5.7063, 3.6643) (5.6998, 3.6621) (5.6934, 3.6599) (5.688, 3.658) (5.6817, 3.6558) (5.6756, 3.6536) (5.6705, 3.6518) (5.6646, 3.6496) (5.6588, 3.6474) (5.6539, 3.6456) (5.6483, 3.6435) (5.6428, 3.6413) (5.6381, 3.6395) (5.6328, 3.6374) (5.6276, 3.6353) (5.6232, 3.6336) (5.6182, 3.6315) (5.6133, 3.6295) (5.6079, 3.6272) (5.6026, 3.625) (5.5974, 3.6227) (5.593, 3.6208) (5.5876, 3.6184) (5.5834, 3.6165) (5.5794, 3.6147) (5.5755, 3.6129) (5.5717, 3.6111) (5.5691, 3.6099) (5.5665, 3.6087) (5.564, 3.6075) (5.5616, 3.6063) (5.5592, 3.6051) (5.5569, 3.604) (5.5546, 3.6029) (5.5524, 3.6018) (5.5503, 3.6007) (5.5482, 3.5996) (5.5462, 3.5986) (5.5442, 3.5976) (5.5424, 3.5966) (5.5405, 3.5957) (5.5388, 3.5947) (5.5371, 3.5938) (5.5355, 3.593) (5.5339, 3.5921) (5.5324, 3.5913) (5.531, 3.5905) (5.5296, 3.5897) (5.5283, 3.589) (5.5271, 3.5883) (5.5259, 3.5877) (5.5248, 3.587) (5.5238, 3.5864) (5.5228, 3.5859) (5.522, 3.5854) (5.5211, 3.5849) (5.5204, 3.5844) (5.5197, 3.584) (5.5191, 3.5837) (5.5185, 3.5833) (5.518, 3.583) (5.5177, 3.5828) (5.5175, 3.5827) (5.5174, 3.5826) knots -1 -1 -1 -1 -1 -1 -0.9875 -0.983333 -0.979167 -0.975 -0.970833 -0.966667 -0.9625 -0.958333 -0.954167 -0.95 -0.945833 -0.941667 -0.9375 -0.933333 -0.929167 -0.925 -0.920833 -0.916667 -0.9125 -0.908333 -0.904167 -0.9 -0.895833 -0.891667 -0.8875 -0.883333 -0.879167 -0.875 -0.870833 -0.866667 -0.854167 -0.85 -0.845833 -0.841667 -0.829167 -0.816667 -0.8125 -0.808333 -0.804167 -0.791667 -0.7875 -0.783333 -0.779167 -0.7625 -0.758333 -0.754167 -0.75 -0.7375 -0.733333 -0.729167 -0.725 -0.7125 -0.708333 -0.704167 -0.7 -0.683333 -0.679167 -0.675 -0.670833 -0.658333 -0.654167 -0.65 -0.645833 -0.633333 -0.629167 -0.625 -0.616667 -0.6125 -0.608333 -0.6 -0.595833 -0.591667 -0.583333 -0.579167 -0.575 -0.566667 -0.5625 -0.558333 -0.55 -0.545833 -0.541667 -0.533333 -0.529167 -0.525 -0.516667 -0.5125 -0.508333 -0.5 -0.495833 -0.491667 -0.483333 -0.479167 -0.475 -0.466667 -0.4625 -0.458333 -0.45 -0.445833 -0.441667 -0.433333 -0.429167 -0.425 -0.416667 -0.4125 -0.408333 -0.4 -0.395833 -0.391667 -0.383333 -0.379167 -0.375 -0.366667 -0.3625 -0.358333 -0.35 -0.345833 -0.341667 -0.333333 -0.329167 -0.325 -0.316667 -0.3125 -0.308333 -0.3 -0.295833 -0.291667 -0.283333 -0.279167 -0.275 -0.266667 -0.2625 -0.258333 -0.25 -0.245833 -0.241667 -0.233333 -0.229167 -0.225 -0.216667 -0.2125 -0.208333 -0.2 -0.195833 -0.183333 -0.179167 -0.175 -0.170833 -0.158333 -0.154167 -0.15 -0.145833 -0.141667 -0.1375 -0.133333 -0.129167 -0.125 -0.120833 -0.116667 -0.1125 -0.108333 -0.104167 -0.1 -0.095833 -0.091667 -0.0875 -0.083333 -0.079167 -0.075 -0.070833 -0.066667 -0.0625 -0.058333 -0.054167 -0.05 -0.045833 -0.041667 -0.0375 -0.033333 -0.029167 -0.025 -0.020833 -0.016667 -0.0125 -0.008333 0 0 0 0 0 0
  arc A25 (7.342, 3.1773) -> (7.0618, 3.7592) centre (0, 0) ccw
  line L50 (6.2404, 2.0798) -> (6.241, 2.08)
  line L51 (5.455, 1.818) -> (6.2404, 2.0798)
  spline S25 degree 5 poles (6.241, 2.08) (6.2411, 2.08) (6.2412, 2.08) (6.2415, 2.0801) (6.2418, 2.0802) (6.2423, 2.0804) (6.2429, 2.0806) (6.2436, 2.0809) (6.2443, 2.0812) (6.2451, 2.0815) (6.246, 2.0818) (6.247, 2.0822) (6.248, 2.0826) (6.2491, 2.083) (6.2503, 2.0835) (6.2515, 2.084) (6.2529, 2.0845) (6.2542, 2.0851) (6.2557, 2.0856) (6.2572, 2.0863) (6.2587, 2.0869) (6.2604, 2.0876) (6.2621, 2.0884) (6.2638, 2.0891) (6.2657, 2.0899) (6.2675, 2.0907) (6.2695, 2.0916) (6.2715, 2.0925) (6.2736, 2.0934) (6.2757, 2.0944) (6.2778, 2.0954) (6.2801, 2.0964) (6.2824, 2.0975) (6.2847, 2.0986) (6.2871, 2.0997) (6.29, 2.1012) (6.2931, 2.1026) (6.2962, 2.1041) (6.3004, 2.1062) (6.3059, 2.109) (6.311, 2.1116) (6.3162, 2.1143) (6.3217, 2.1172) (6.3279, 2.1205) (6.333, 2.1232) (6.3382, 2.1261) (6.3435, 2.129) (6.3503, 2.1328) (6.3551, 2.1356) (6.3601, 2.1384) (6.3651, 2.1413) (6.3724, 2.1456) (6.3783, 2.1491) (6.3844, 2.1528) (6.3905, 2.1565) (6.3984, 2.1613) (6.4039, 2.1648) (6.4095, 2.1683) (6.4152, 2.1719) (6.4226, 2.1767) (6.4285, 2.1805) (6.4344, 2.1843) (6.4404, 2.1883) (6.449, 2.194) (6.456, 2.1987) (6.4631, 2.2035) (6.4702, 2.2085) (6.4792, 2.2148) (6.4856, 2.2192) (6.4921, 2.2238) (6.4986, 2.2285) (6.507, 2.2346) (6.5136, 2.2394) (6.5203, 2.2443) (6.527, 2.2493) (6.5357, 2.2558) (6.5426, 2.261) (6.5494, 2.2662) (6.5573, 2.2723) (6.5653, 2.2785) (6.5713, 2.2832) (6.5774, 2.288) (6.5855, 2.2944) (6.5926, 2.3001) (6.5998, 2.3059) (6.608, 2.3126) (6.6163, 2.3195) (6.6226, 2.3246) (6.6299, 2.3308) (6.6373, 2.337) (6.6436, 2.3423) (6.651, 2.3487) (6.6585, 2.3551) (6.6649, 2.3607) (6.6724, 2.3672) (6.68, 2.3739) (6.6865, 2.3797) (6.6941, 2.3864) (6.7017, 2.3933) (6.7083, 2.3993) (6.716, 2.4063) (6.7237, 2.4134) (6.7304, 2.4195) (6.7381, 2.4268) (6.7459, 2.4341) (6.7526, 2.4404) (6.7604, 2.4479) (6.7683, 2.4554) (6.775, 2.4619) (6.7829, 2.4696) (6.7908, 2.4774) (6.7977, 2.4841) (6.8056, 2.492) (6.8136, 2.5) (6.8204, 2.5069) (6.8284, 2.515) (6.8364, 2.5232) (6.8433, 2.5303) (6.8514, 2.5387) (6.8595, 2.5471) (6.8664, 2.5544) (6.8745, 2.5629) (6.8826, 2.5716) (6.8895, 2.5791) (6.8977, 2.5878) (6.9058, 2.5967) (6.9128, 2.6044) (6.921, 2.6134) (6.9291, 2.6225) (6.9362, 2.6303) (6.9443, 2.6395) (6.9525, 2.6488) (6.9596, 2.6569) (6.9678, 2.6663) (6.976, 2.6758) (6.983, 2.684) (6.9925, 2.6951) (7.0019, 2.7062) (7.0101, 2.7161) (7.0195, 2.7274) (7.029, 2.7388) (7.036, 2.7475) (7.0443, 2.7576) (7.0525, 2.7678) (7.0596, 2.7766) (7.0679, 2.787) (7.0761, 2.7974) (7.0832, 2.8064) (7.0903, 2.8155) (7.0985, 2.8261) (7.1056, 2.8353) (7.1127, 2.8445) (7.1197, 2.8538) (7.1268, 2.8632) (7.1339, 2.8726) (7.1409, 2.882) (7.1492, 2.8931) (7.1574, 2.9042) (7.1656, 2.9155) (7.1727, 2.9252) (7.1797, 2.9349) (7.1856, 2.9431) (7.1914, 2.9513) (7.1973, 2.9595) (7.2031, 2.9678) (7.209, 2.9761) (7.2148, 2.9844) (7.2207, 2.9928) (7.2265, 3.0012) (7.2323, 3.0097) (7.2381, 3.0182) (7.244, 3.0267) (7.2498, 3.0353) (7.2556, 3.0439) (7.2614, 3.0525) (7.2672, 3.0612) (7.273, 3.0699) (7.2788, 3.0787) (7.2846, 3.0875) (7.2903, 3.0963) (7.2961, 3.1051) (7.3019, 3.114) (7.3076, 3.123) (7.3168, 3.1373) (7.3248, 3.15) (7.3317, 3.1609) (7.3374, 3.17) (7.342, 3.1773) knots 0 0 0 0 0 0 0.004167 0.008333 0.0125 0.016667 0.020833 0.025 0.029167 0.033333 0.0375 0.041667 0.045833 0.05 0.054167 0.058333 0.0625 0.066667 0.070833 0.075 0.079167 0.083333 0.0875 0.091667 0.095833 0.1 0.104167 0.108333 0.1125 0.116667 0.120833 0.125 0.129167 0.133333 0.1375 0.141667 0.15 0.154167 0.158333 0.170833 0.183333 0.1875 0.191667 0.195833 0.2125 0.216667 0.220833 0.225 0.2375 0.241667 0.245833 0.25 0.266667 0.270833 0.275 0.279167 0.291667 0.295833 0.3 0.304167 0.316667 0.320833 0.325 0.329167 0.345833 0.35 0.354167 0.358333 0.370833 0.375 0.379167 0.383333 0.395833 0.4 0.404167 0.408333 0.420833 0.425 0.429167 0.4375 0.441667 0.445833 0.45 0.4625 0.466667 0.470833 0.479167 0.483333 0.4875 0.495833 0.5 0.504167 0.5125 0.516667 0.520833 0.529167 0.533333 0.5375 0.545833 0.55 0.554167 0.5625 0.566667 0.570833 0.579167 0.583333 0.5875 0.595833 0.6 0.604167 0.6125 0.616667 0.620833 0.629167 0.633333 0.6375 0.645833 0.65 0.654167 0.6625 0.666667 0.670833 0.679167 0.683333 0.6875 0.695833 0.7 0.704167 0.7125 0.716667 0.720833 0.729167 0.733333 0.7375 0.745833 0.75 0.754167 0.766667 0.770833 0.775 0.783333 0.7875 0.791667 0.8 0.804167 0.808333 0.816667 0.820833 0.825 0.829167 0.8375 0.841667 0.845833 0.85 0.854167 0.8625 0.866667 0.875 0.879167 0.883333 0.8875 0.891667 0.895833 0.9 0.904167 0.908333 0.9125 0.916667 0.920833 0.925 0.929167 0.933333 0.9375 0.941667 0.945833 0.95 0.954167 0.958333 0.9625 0.966667 0.970833 0.975 0.979167 0.983333 1 1 1 1 1 1
  arc A26 (5.7036, 0.7289) -> (5.455, 1.818) centre (0, 0) ccw
  line L52 (6.5254, 0.8339) -> (6.5248, 0.8338)
  line L53 (5.7036, -0.7289) -> (6.5248, -0.8338)
  line L54 (6.5248, -0.8338) -> (6.5254, -0.8339)
  spline S26 degree 5 poles (7.9935, 0.3229) (7.988, 0.3264) (7.9807, 0.331) (7.9716, 0.3367) (7.9607, 0.3435) (7.948, 0.3514) (7.9389, 0.357) (7.9299, 0.3625) (7.9208, 0.368) (7.9118, 0.3735) (7.9028, 0.3789) (7.8937, 0.3843) (7.8847, 0.3897) (7.8757, 0.3951) (7.8667, 0.4004) (7.8578, 0.4056) (7.8488, 0.4109) (7.8398, 0.4161) (7.8309, 0.4212) (7.822, 0.4263) (7.813, 0.4314) (7.8041, 0.4365) (7.7952, 0.4415) (7.7863, 0.4465) (7.7775, 0.4514) (7.7686, 0.4563) (7.7598, 0.4612) (7.7509, 0.4661) (7.7421, 0.4709) (7.7333, 0.4756) (7.7227, 0.4813) (7.7122, 0.487) (7.7017, 0.4925) (7.6912, 0.4981) (7.6772, 0.5054) (7.665, 0.5117) (7.6529, 0.5179) (7.6408, 0.5241) (7.6252, 0.5319) (7.6131, 0.538) (7.6011, 0.5439) (7.5891, 0.5498) (7.5737, 0.5573) (7.5618, 0.563) (7.5499, 0.5687) (7.5364, 0.5751) (7.5229, 0.5814) (7.5128, 0.586) (7.501, 0.5914) (7.4893, 0.5967) (7.4793, 0.6013) (7.4677, 0.6065) (7.4561, 0.6116) (7.4462, 0.6159) (7.4346, 0.6209) (7.4231, 0.6259) (7.4133, 0.6301) (7.4019, 0.6349) (7.3905, 0.6397) (7.3808, 0.6437) (7.3695, 0.6483) (7.3582, 0.6529) (7.3486, 0.6568) (7.3374, 0.6612) (7.3263, 0.6656) (7.3168, 0.6693) (7.3057, 0.6736) (7.2947, 0.6778) (7.2853, 0.6814) (7.2744, 0.6855) (7.2635, 0.6895) (7.2542, 0.6929) (7.2434, 0.6968) (7.2327, 0.7006) (7.2235, 0.7039) (7.2129, 0.7076) (7.2023, 0.7113) (7.1932, 0.7144) (7.1827, 0.718) (7.1723, 0.7215) (7.1634, 0.7244) (7.153, 0.7278) (7.1427, 0.7311) (7.134, 0.7339) (7.1238, 0.7371) (7.1136, 0.7403) (7.105, 0.7429) (7.095, 0.746) (7.085, 0.749) (7.0765, 0.7515) (7.0666, 0.7544) (7.0568, 0.7572) (7.0485, 0.7595) (7.0388, 0.7623) (7.0292, 0.7649) (7.021, 0.7671) (7.0114, 0.7697) (7.002, 0.7722) (6.9939, 0.7743) (6.9846, 0.7767) (6.9754, 0.779) (6.9675, 0.781) (6.9583, 0.7832) (6.9493, 0.7854) (6.9416, 0.7872) (6.9326, 0.7893) (6.9237, 0.7913) (6.9162, 0.793) (6.9075, 0.7949) (6.8988, 0.7968) (6.8914, 0.7984) (6.8829, 0.8002) (6.8744, 0.8019) (6.8673, 0.8033) (6.8589, 0.805) (6.8507, 0.8066) (6.8437, 0.8079) (6.8356, 0.8094) (6.8276, 0.8108) (6.8208, 0.812) (6.8129, 0.8134) (6.8052, 0.8147) (6.7986, 0.8158) (6.7909, 0.8171) (6.7834, 0.8182) (6.777, 0.8192) (6.7696, 0.8203) (6.7623, 0.8214) (6.7561, 0.8223) (6.749, 0.8232) (6.7419, 0.8242) (6.736, 0.8249) (6.7291, 0.8258) (6.7223, 0.8266) (6.7166, 0.8273) (6.7099, 0.828) (6.7034, 0.8287) (6.6979, 0.8293) (6.6916, 0.83) (6.6853, 0.8306) (6.6801, 0.8311) (6.674, 0.8316) (6.668, 0.8321) (6.663, 0.8325) (6.6573, 0.8329) (6.6516, 0.8333) (6.6468, 0.8337) (6.6406, 0.8341) (6.6345, 0.8344) (6.6292, 0.8347) (6.6241, 0.8349) (6.617, 0.8353) (6.6115, 0.8355) (6.6061, 0.8356) (6.6009, 0.8358) (6.5959, 0.8359) (6.5922, 0.836) (6.5885, 0.836) (6.585, 0.836) (6.5816, 0.8361) (6.5782, 0.8361) (6.5755, 0.8361) (6.5729, 0.8361) (6.5703, 0.836) (6.5678, 0.836) (6.5653, 0.836) (6.5629, 0.8359) (6.5606, 0.8359) (6.5583, 0.8358) (6.5561, 0.8358) (6.554, 0.8357) (6.5519, 0.8356) (6.55, 0.8356) (6.548, 0.8355) (6.5462, 0.8354) (6.5444, 0.8353) (6.5427, 0.8352) (6.5411, 0.8351) (6.5395, 0.835) (6.5381, 0.8349) (6.5366, 0.8349) (6.5353, 0.8348) (6.5341, 0.8347) (6.5329, 0.8346) (6.5318, 0.8345) (6.5307, 0.8344) (6.5298, 0.8343) (6.5289, 0.8343) (6.5281, 0.8342) (6.5274, 0.8341) (6.5267, 0.834) (6.5262, 0.834) (6.5258, 0.8339) (6.5256, 0.8339) (6.5254, 0.8339) knots -1 -1 -1 -1 -1 -1 -0.9875 -0.983333 -0.979167 -0.975 -0.970833 -0.966667 -0.9625 -0.958333 -0.954167 -0.95 -0.945833 -0.941667 -0.9375 -0.933333 -0.929167 -0.925 -0.920833 -0.916667 -0.9125 -0.908333 -0.904167 -0.9 -0.895833 -0.891667 -0.8875 -0.883333 -0.879167 -0.875 -0.870833 -0.8625 -0.858333 -0.854167 -0.85 -0.8375 -0.833333 -0.829167 -0.825 -0.8125 -0.808333 -0.804167 -0.8 -0.7875 -0.783333 -0.779167 -0.770833 -0.766667 -0.7625 -0.754167 -0.75 -0.745833 -0.7375 -0.733333 -0.729167 -0.720833 -0.716667 -0.7125 -0.704167 -0.7 -0.695833 -0.6875 -0.683333 -0.679167 -0.670833 -0.666667 -0.6625 -0.654167 -0.65 -0.645833 -0.6375 -0.633333 -0.629167 -0.620833 -0.616667 -0.6125 -0.604167 -0.6 -0.595833 -0.5875 -0.583333 -0.579167 -0.570833 -0.566667 -0.5625 -0.554167 -0.55 -0.545833 -0.5375 -0.533333 -0.529167 -0.520833 -0.516667 -0.5125 -0.504167 -0.5 -0.495833 -0.4875 -0.483333 -0.479167 -0.470833 -0.466667 -0.4625 -0.454167 -0.45 -0.445833 -0.4375 -0.433333 -0.429167 -0.420833 -0.416667 -0.4125 -0.404167 -0.4 -0.395833 -0.3875 -0.383333 -0.379167 -0.370833 -0.366667 -0.3625 -0.354167 -0.35 -0.345833 -0.3375 -0.333333 -0.329167 -0.320833 -0.316667 -0.3125 -0.304167 -0.3 -0.295833 -0.2875 -0.283333 -0.279167 -0.270833 -0.266667 -0.2625 -0.254167 -0.25 -0.245833 -0.2375 -0.233333 -0.229167 -0.220833 -0.216667 -0.2125 -0.2 -0.195833 -0.191667 -0.1875 -0.170833 -0.166667 -0.1625 -0.158333 -0.154167 -0.145833 -0.141667 -0.1375 -0.133333 -0.129167 -0.125 -0.120833 -0.116667 -0.1125 -0.108333 -0.104167 -0.1 -0.095833 -0.091667 -0.0875 -0.083333 -0.079167 -0.075 -0.070833 -0.066667 -0.0625 -0.058333 -0.054167 -0.05 -0.045833 -0.041667 -0.0375 -0.033333 -0.029167 -0.025 -0.020833 -0.016667 -0.0125 -0.008333 0 0 0 0 0 0
  arc A27 (7.9935, -0.3229) -> (7.9935, 0.3229) centre (0, 0) ccw